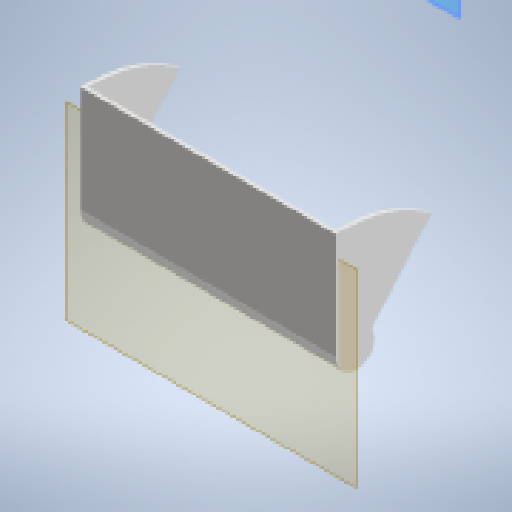
# Autodesk Inventor part: 앞문
Saved by Autodesk Inventor 2025 (Build 290162010, 162A)
## iProperties
Created: 2024-05-29
Part Number: 앞문
Material: 일반
Document SubType Name: Modeling
Designer: user
Density: 1 g/cm^3
Appearance: 기본값
Author: user
Autodesk Inventor part; units mm, degrees
ref_plane "YZ Plane" through (0, 0, 0) normal (1, 0, 0) x (0, 1, 0)
ref_plane "XZ Plane" through (0, 0, 0) normal (0, 1, 0) x (-1, 0, 0)
ref_plane "XY Plane" through (0, 0, 0) normal (0, 0, 1) x (1, 0, 0)
ref_plane "작업 평면1" through (0, 0.7157, 0) normal (0, 0, 1) x (1, 0, 0)
sketch "스케치1" plane through (0, 0.7157, 0) normal (0, 0, 1) x (1, 0, 0)
  line L0 (70.0112, 388.9292) -> (730.0112, 388.9292)
  line L1 (730.0112, 388.9292) -> (730.0112, 718.9292)
  line L2 (730.0112, 718.9292) -> (70.0112, 718.9292)
  line L3 (70.0112, 718.9292) -> (70.0112, 388.9292)
  point P0 (0, -0.7157)
  dimension "d0" = 660
  dimension "d1" = 330
  constraints: 8 end point, 2 parallel, 1 horizontal, 1 perpendicular
  measures "d0" distance of L2.end L1.end
  measures "d1" distance of L1.end L0.end
extrude "돌출1" add sketch "스케치1" along normal blind 10
sketch "스케치2" plane through (0, 0.7157, 0) normal (0, 0, -1) x (-1, 0, 0)
  line L0 (-70.0112, 388.9292) -> (-730.0112, 388.9292) projected
  line L1 (-730.0112, 388.9292) -> (-720.0112, 388.9292)
  line L2 (-720.0112, 388.9292) -> (-720.0112, 478.9292)
  line L3 (-720.0112, 478.9292) -> (-730.0112, 478.9292)
  line L4 (-730.0112, 478.9292) -> (-730.0112, 388.9292)
  line L5 (-70.0112, 388.9292) -> (-80.0112, 388.9292)
  line L6 (-80.0112, 388.9292) -> (-80.0112, 478.9292)
  line L7 (-80.0112, 478.9292) -> (-70.0112, 478.9292)
  line L8 (-70.0112, 478.9292) -> (-70.0112, 388.9292)
  point P0 (0, -0.7157)
  dimension "d4" = 10
  dimension "d5" = 90
  dimension "d6" = 10
  dimension "d7" = 90
  constraints: 16 end point, 4 parallel, 2 horizontal, 2 perpendicular
  measures "d4" distance of L3.end L2.end
  measures "d5" distance of L2.end L1.end
  measures "d6" distance of L6.end L7.end
  measures "d7" distance of L5.end L6.end
extrude "돌출2" add sketch "스케치2" along normal blind 90
fillet "모깎기1" radius 45 4 edges at (725.0112, 479.645, -90) (725.0112, 389.645, -90) (75.0112, 479.645, -90) (75.0112, 389.645, -90)
fillet "모깎기2" radius 55 1 edges at (400.0112, 389.645, 10)
sketch "스케치3" plane through (730.0112, 719.645, 10) normal (1, 0, 0) x (0, 0, -1)
  line L0 (10, -240) -> (10, 0) projected
  arc A0 (247.7061, -77.4327) -> (10, 0) centre (14.4307, -389.9748) ccw
  line L1 (10, 0) -> (10, -240)
  line L2 (247.7061, -77.4327) -> (91.8862, -259.2239)
  arc A1 (55, -330) -> (55, -240) centre (55, -285) ccw projected
  line L3 (10, -240) -> (55, -240) projected
  line L4 (10, -240) -> (55, -240)
  arc A2 (91.8862, -259.2239) -> (55, -240) centre (55, -285) ccw
  point P0 (10, -719.645)
  dimension "d12" = 250
  dimension "d13" = 390
  constraints: 6 end point, 6 point on circle, 2 centre point, 2 collinear, 1 concentric
  measures "d12" distance of L0.end L2.start
  measures "d13" radius of A0
extrude "돌출3" add sketch "스케치3" against normal blind 10
sketch "스케치4" plane through (70.0112, 719.645, 0) normal (-1, 0, 0) x (0, 0, 1)
  line L0 (-237.7061, -77.4327) -> (-81.8862, -259.2239) projected
  line L1 (-237.7061, -77.4327) -> (-81.8862, -259.2239)
  line L2 (0, 0) -> (10, 0) projected
  arc A0 (0, 0) -> (-237.7061, -77.4327) centre (-4.4307, -389.9748) ccw
  line L3 (0, 0) -> (0, -240) projected
  line L4 (0, 0) -> (0, -240)
  arc A1 (-45, -240) -> (-45, -330) centre (-45, -285) ccw projected
  line L5 (0, -240) -> (-45, -240)
  arc A2 (-45, -240) -> (-81.8862, -259.2239) centre (-45, -285) ccw
  point P0 (0, -719.645)
  constraints: 6 end point, 4 point on circle, 2 centre point, 1 collinear, 1 concentric, 1 perpendicular, 1 tangent, 1 vertical
extrude "돌출4" add sketch "스케치4" against normal blind 10
sketch "스케치5" plane through (730.0112, 444.645, 10) normal (1, 0, 0) x (0, 0, -1)
  arc A0 (55, -55) -> (91.8862, 15.7761) centre (55, -10) ccw projected
  circle A1 centre (55, -10) radius 5
  point P0 (10, -444.645)
  dimension "d18" = 10
  constraints: 1 centre point, 1 coincident
  measures "d18" diameter of A1
extrude "돌출5" add sketch "스케치5" along normal blind 10
sketch "스케치6" plane through (70.0112, 444.645, 10) normal (-1, 0, 0) x (0, 0, 1)
  arc A0 (-91.8862, 15.7761) -> (-55, -55) centre (-55, -10) ccw projected
  circle A1 centre (-55, -10) radius 5
  point P0 (-10, -444.645)
  constraints: 1 centre point, 1 coincident
extrude "돌출6" add sketch "스케치6" along normal blind 10
